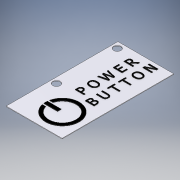
# Autodesk Inventor part: Power Button Plate
Saved by Autodesk Inventor 2019 (Build 230136000, 136)
## iProperties
Created: 2019-02-07
Part Number: Power Button Plate
Material: Generic
Document SubType Name: Modeling
Designer: mrhftc
Density: 1 g/cm^3
Appearance: Default
Author: mrhftc
Autodesk Inventor part; units mm, degrees
ref_plane "YZ Plane" through (0, 0, 0) normal (1, 0, 0) x (0, 1, 0)
ref_plane "XZ Plane" through (0, 0, 0) normal (0, 1, 0) x (-1, 0, 0)
ref_plane "XY Plane" through (0, 0, 0) normal (0, 0, 1) x (1, 0, 0)
sketch "Sketch1" plane through (0, 0, 0) normal (0, 1, 0) x (-1, 0, 0)
  line L0 (9.9313, 40.7784) -> (41.6813, 40.7784)
  line L1 (41.6813, 40.7784) -> (41.6813, 104.2784)
  line L2 (41.6813, 104.2784) -> (9.9313, 104.2784)
  line L3 (9.9313, 104.2784) -> (9.9313, 40.7784)
  point P0 (0, 0)
  dimension "d0" = 63.5
  dimension "d1" = 31.75
  constraints: 8 end point, 2 parallel, 1 horizontal, 1 perpendicular
  measures "d0" distance between parallel lines of L0 L2
  measures "d1" distance between parallel lines of L3 L1
extrude "Extrusion1" add sketch "Sketch1" along normal blind 0.3175
sketch "Sketch2" plane through (0, 0.3175, 0) normal (0, 1, 0) x (1, 0, 0)
  line L0 (-9.9313, -40.7784) -> (-41.6813, -40.7784) construction
  line L1 (-41.6813, -40.7784) -> (-41.6813, -104.2784) construction
  line L2 (-9.9313, -104.2784) -> (-9.9313, -40.7784) construction
  line L3 (-9.9313, -104.2784) -> (-35.3313, -104.2784)
  line L4 (-35.3313, -104.2784) -> (-35.3313, -40.7784)
  line L5 (-35.3313, -40.7784) -> (-9.9313, -40.7784)
  line L6 (-9.9313, -40.7784) -> (-9.9313, -104.2784)
  circle A0 centre (-38.5063, -44.3234) radius 2.1
  circle A1 centre (-38.5063, -78.8784) radius 2.1
  arc A2 (-32.0131, -93.4738) -> (-32.0131, -89.3044) centre (-22.6313, -91.3891) ccw
  arc A3 (-30.0496, -93.4738) -> (-30.0496, -89.3044) centre (-22.6313, -91.3891) ccw
  line L7 (-32.2013, -92.4142) -> (-24.3428, -92.4142)
  line L8 (-24.3428, -92.4142) -> (-24.3428, -90.3641)
  line L9 (-24.3428, -90.3641) -> (-32.2013, -90.3641)
  line L10 (-32.2013, -90.3641) -> (-32.2013, -92.4142)
  line L11 (-32.0131, -93.4738) -> (-30.0496, -93.4738)
  line L12 (-32.0131, -89.3044) -> (-30.0496, -89.3044)
  line L13 (-31.0313, -79.4258) -> (-24.997, -79.4258)
  line L14 (-24.997, -79.4258) -> (-24.997, -43.023)
  line L15 (-24.997, -43.023) -> (-31.0313, -43.023)
  line L16 (-31.0313, -43.023) -> (-31.0313, -79.4258)
  spline S0 degree 2 poles (-28.5456, -73.5374) (-28.2163, -73.5374) (-27.6235, -73.7721) (-27.4176, -73.982) knots 0 0 0 1 2 2 2
  spline S1 degree 2 poles (-27.4176, -73.982) (-27.1583, -74.2455) (-26.8907, -74.9577) (-26.8907, -75.5011) knots 0 0 0 1 2 2 2
  line L17 (-26.8907, -75.5011) -> (-26.8907, -76.0733)
  line L18 (-26.8907, -76.0733) -> (-24.997, -76.0733)
  line L19 (-24.997, -76.0733) -> (-24.997, -76.7485)
  line L20 (-24.997, -76.7485) -> (-30.077, -76.7485)
  line L21 (-30.077, -76.7485) -> (-30.077, -75.4723)
  spline S2 degree 2 poles (-30.077, -75.4723) (-30.077, -75.0194) (-29.9288, -74.3855) (-29.76, -74.1426) knots 0 0 0 1 2 2 2
  spline S3 degree 2 poles (-29.76, -74.1426) (-29.5665, -73.8585) (-28.9696, -73.5374) (-28.5456, -73.5374) knots 0 0 0 1 2 2 2
  spline S4 degree 2 poles (-28.525, -74.2414) (-28.7885, -74.2414) (-29.1754, -74.4225) (-29.2989, -74.6078) knots 0 0 0 1 2 2 2
  spline S5 degree 2 poles (-29.2989, -74.6078) (-29.406, -74.7683) (-29.4924, -75.1965) (-29.4924, -75.5134) knots 0 0 0 1 2 2 2
  line L22 (-29.4924, -75.5134) -> (-29.4924, -76.0733)
  line L23 (-29.4924, -76.0733) -> (-27.467, -76.0733)
  line L24 (-27.467, -76.0733) -> (-27.467, -75.6122)
  spline S6 degree 2 poles (-27.467, -75.6122) (-27.467, -75.2006) (-27.5988, -74.6942) (-27.7717, -74.5296) knots 0 0 0 1 2 2 2
  spline S7 degree 2 poles (-27.7717, -74.5296) (-27.924, -74.3772) (-28.2821, -74.2414) (-28.525, -74.2414) knots 0 0 0 1 2 2 2
  spline S8 degree 2 poles (-29.4965, -67.1195) (-29.159, -66.8313) (-28.171, -66.5102) (-27.537, -66.5102) knots 0 0 0 1 2 2 2
  spline S9 degree 2 poles (-27.537, -66.5102) (-26.9195, -66.5102) (-25.9191, -66.8231) (-25.5816, -67.1195) knots 0 0 0 1 2 2 2
  spline S10 degree 2 poles (-25.5816, -67.1195) (-25.2275, -67.4324) (-24.89, -68.2598) (-24.89, -68.758) knots 0 0 0 1 2 2 2
  spline S11 degree 2 poles (-24.89, -68.758) (-24.89, -69.2725) (-25.2399, -70.0959) (-25.5816, -70.3964) knots 0 0 0 1 2 2 2
  spline S12 degree 2 poles (-25.5816, -70.3964) (-25.9191, -70.6887) (-26.9113, -71.0016) (-27.537, -71.0016) knots 0 0 0 1 2 2 2
  spline S13 degree 2 poles (-27.537, -71.0016) (-28.1751, -71.0016) (-29.1466, -70.6846) (-29.4965, -70.3923) knots 0 0 0 1 2 2 2
  spline S14 degree 2 poles (-29.4965, -70.3923) (-29.8341, -70.0959) (-30.184, -69.2684) (-30.184, -68.758) knots 0 0 0 1 2 2 2
  spline S15 degree 2 poles (-30.184, -68.758) (-30.184, -68.2392) (-29.8218, -67.4077) (-29.4965, -67.1195) knots 0 0 0 1 2 2 2
  spline S16 degree 2 poles (-27.537, -67.2142) (-28.0392, -67.2142) (-28.8173, -67.4324) (-29.0725, -67.63) knots 0 0 0 1 2 2 2
  spline S17 degree 2 poles (-29.0725, -67.63) (-29.336, -67.8317) (-29.5995, -68.3998) (-29.5995, -68.7538) knots 0 0 0 1 2 2 2
  spline S18 degree 2 poles (-29.5995, -68.7538) (-29.5995, -69.1202) (-29.3442, -69.6719) (-29.0725, -69.8818) knots 0 0 0 1 2 2 2
  spline S19 degree 2 poles (-29.0725, -69.8818) (-28.8132, -70.0835) (-28.031, -70.2976) (-27.537, -70.2976) knots 0 0 0 1 2 2 2
  spline S20 degree 2 poles (-27.537, -70.2976) (-26.5366, -70.2976) (-25.4745, -69.4578) (-25.4745, -68.7538) knots 0 0 0 1 2 2 2
  spline S21 degree 2 poles (-25.4745, -68.7538) (-25.4745, -68.0499) (-26.5366, -67.2142) (-27.537, -67.2142) knots 0 0 0 1 2 2 2
  line L25 (-30.077, -57.894) -> (-24.997, -59.1702)
  line L26 (-24.997, -59.1702) -> (-24.997, -59.9276)
  line L27 (-24.997, -59.9276) -> (-29.2125, -60.9609)
  line L28 (-29.2125, -60.9609) -> (-24.997, -61.9654)
  line L29 (-24.997, -61.9654) -> (-24.997, -62.7146)
  line L30 (-24.997, -62.7146) -> (-30.077, -64.0114)
  line L31 (-30.077, -64.0114) -> (-30.077, -63.3157)
  line L32 (-30.077, -63.3157) -> (-25.8656, -62.2947)
  line L33 (-25.8656, -62.2947) -> (-30.077, -61.282)
  line L34 (-30.077, -61.282) -> (-30.077, -60.5945)
  line L35 (-30.077, -60.5945) -> (-25.8162, -59.5736)
  line L36 (-25.8162, -59.5736) -> (-30.077, -58.5568)
  line L37 (-30.077, -58.5568) -> (-30.077, -57.894)
  line L38 (-24.997, -55.107) -> (-30.077, -55.107)
  line L39 (-30.077, -55.107) -> (-30.077, -51.9289)
  line L40 (-30.077, -51.9289) -> (-29.476, -51.9289)
  line L41 (-29.476, -51.9289) -> (-29.476, -54.4319)
  line L42 (-29.476, -54.4319) -> (-28.0845, -54.4319)
  line L43 (-28.0845, -54.4319) -> (-28.0845, -52.0977)
  line L44 (-28.0845, -52.0977) -> (-27.4835, -52.0977)
  line L45 (-27.4835, -52.0977) -> (-27.4835, -54.4319)
  line L46 (-27.4835, -54.4319) -> (-25.598, -54.4319)
  line L47 (-25.598, -54.4319) -> (-25.598, -51.9289)
  line L48 (-25.598, -51.9289) -> (-24.997, -51.9289)
  line L49 (-24.997, -51.9289) -> (-24.997, -55.107)
  line L50 (-24.997, -45.0746) -> (-24.997, -45.9515)
  line L51 (-24.997, -45.9515) -> (-27.0183, -47.557)
  line L52 (-27.0183, -47.557) -> (-27.0183, -48.3309)
  line L53 (-27.0183, -48.3309) -> (-24.997, -48.3309)
  line L54 (-24.997, -48.3309) -> (-24.997, -49.0061)
  line L55 (-24.997, -49.0061) -> (-30.077, -49.0061)
  line L56 (-30.077, -49.0061) -> (-30.077, -47.6969)
  spline S22 degree 2 poles (-30.077, -47.6969) (-30.077, -47.2606) (-29.9823, -46.6719) (-29.8094, -46.4043) knots 0 0 0 1 2 2 2
  spline S23 degree 2 poles (-29.8094, -46.4043) (-29.6365, -46.1367) (-29.0972, -45.828) (-28.6979, -45.828) knots 0 0 0 1 2 2 2
  spline S24 degree 2 poles (-28.6979, -45.828) (-28.1422, -45.828) (-27.3888, -46.3961) (-27.2077, -46.8818) knots 0 0 0 1 2 2 2
  line L57 (-27.2077, -46.8818) -> (-24.997, -45.0746)
  spline S25 degree 2 poles (-28.6444, -46.5319) (-28.8667, -46.5319) (-29.2084, -46.6884) (-29.3195, -46.853) knots 0 0 0 1 2 2 2
  spline S26 degree 2 poles (-29.3195, -46.853) (-29.4142, -46.9971) (-29.4924, -47.38) (-29.4924, -47.6599) knots 0 0 0 1 2 2 2
  line L58 (-29.4924, -47.6599) -> (-29.4924, -48.3309)
  line L59 (-29.4924, -48.3309) -> (-27.5823, -48.3309)
  line L60 (-27.5823, -48.3309) -> (-27.5823, -47.7381)
  spline S27 degree 2 poles (-27.5823, -47.7381) (-27.5823, -47.4458) (-27.6852, -46.9806) (-27.8458, -46.8201) knots 0 0 0 1 2 2 2
  spline S28 degree 2 poles (-27.8458, -46.8201) (-27.9857, -46.6719) (-28.3809, -46.5319) (-28.6444, -46.5319) knots 0 0 0 1 2 2 2
  spline S29 degree 2 poles (-18.1683, -75.9519) (-17.7896, -75.9519) (-17.2091, -76.24) (-17.0198, -76.4788) knots 0 0 0 1 2 2 2
  spline S30 degree 2 poles (-17.0198, -76.4788) (-16.7975, -76.767) (-16.6081, -77.4215) (-16.6081, -77.9402) knots 0 0 0 1 2 2 2
  line L61 (-16.6081, -77.9402) -> (-16.6081, -79.3975)
  line L62 (-16.6081, -79.3975) -> (-21.6881, -79.3975)
  line L63 (-21.6881, -79.3975) -> (-21.6881, -78.0514)
  spline S31 degree 2 poles (-21.6881, -78.0514) (-21.6881, -77.508) (-21.6181, -76.9646) (-21.4823, -76.7176) knots 0 0 0 1 2 2 2
  spline S32 degree 2 poles (-21.4823, -76.7176) (-21.3382, -76.4418) (-20.8648, -76.1906) (-20.5437, -76.1906) knots 0 0 0 1 2 2 2
  spline S33 degree 2 poles (-20.5437, -76.1906) (-20.1855, -76.1906) (-19.6174, -76.5694) (-19.4569, -76.9028) knots 0 0 0 1 2 2 2
  line L64 (-19.4569, -76.9028) -> (-19.4322, -76.9028)
  spline S34 degree 2 poles (-19.4322, -76.9028) (-19.3086, -76.45) (-18.6541, -75.9519) (-18.1683, -75.9519) knots 0 0 0 1 2 2 2
  spline S35 degree 2 poles (-18.1395, -76.6558) (-18.4277, -76.6558) (-18.7982, -76.8205) (-18.9299, -77.0675) knots 0 0 0 1 2 2 2
  spline S36 degree 2 poles (-18.9299, -77.0675) (-19.0122, -77.2281) (-19.0616, -77.6068) (-19.0616, -77.9567) knots 0 0 0 1 2 2 2
  line L65 (-19.0616, -77.9567) -> (-19.0616, -78.7224)
  line L66 (-19.0616, -78.7224) -> (-17.1844, -78.7224)
  line L67 (-17.1844, -78.7224) -> (-17.1844, -78.1749)
  spline S37 degree 2 poles (-17.1844, -78.1749) (-17.1844, -77.7303) (-17.2668, -77.2198) (-17.3985, -77.0222) knots 0 0 0 1 2 2 2
  spline S38 degree 2 poles (-17.3985, -77.0222) (-17.5344, -76.8328) (-17.8719, -76.6558) (-18.1395, -76.6558) knots 0 0 0 1 2 2 2
  spline S39 degree 2 poles (-20.449, -76.8946) (-20.6301, -76.8946) (-20.9018, -77.0181) (-20.98, -77.1539) knots 0 0 0 1 2 2 2
  spline S40 degree 2 poles (-20.98, -77.1539) (-21.0706, -77.3186) (-21.1118, -77.7179) (-21.1118, -78.0761) knots 0 0 0 1 2 2 2
  line L68 (-21.1118, -78.0761) -> (-21.1118, -78.7224)
  line L69 (-21.1118, -78.7224) -> (-19.6256, -78.7224)
  line L70 (-19.6256, -78.7224) -> (-19.6256, -77.9567)
  spline S41 degree 2 poles (-19.6256, -77.9567) (-19.6256, -77.6397) (-19.6915, -77.3392) (-19.7944, -77.1787) knots 0 0 0 1 2 2 2
  spline S42 degree 2 poles (-19.7944, -77.1787) (-19.8932, -77.0222) (-20.2102, -76.8946) (-20.449, -76.8946) knots 0 0 0 1 2 2 2
  spline S43 degree 2 poles (-16.5011, -71.3247) (-16.5011, -71.7734) (-16.7357, -72.4403) (-16.9704, -72.675) knots 0 0 0 1 2 2 2
  spline S44 degree 2 poles (-16.9704, -72.675) (-17.2338, -72.9426) (-17.9748, -73.1608) (-18.5182, -73.1608) knots 0 0 0 1 2 2 2
  line L71 (-18.5182, -73.1608) -> (-21.6881, -73.1608)
  line L72 (-21.6881, -73.1608) -> (-21.6881, -72.4856)
  line L73 (-21.6881, -72.4856) -> (-18.5182, -72.4856)
  spline S45 degree 2 poles (-18.5182, -72.4856) (-18.1642, -72.4856) (-17.6867, -72.3951) (-17.4932, -72.2674) knots 0 0 0 1 2 2 2
  spline S46 degree 2 poles (-17.4932, -72.2674) (-17.2874, -72.1316) (-17.0774, -71.6623) (-17.0774, -71.3247) knots 0 0 0 1 2 2 2
  spline S47 degree 2 poles (-17.0774, -71.3247) (-17.0774, -71.0077) (-17.2874, -70.5137) (-17.4932, -70.3779) knots 0 0 0 1 2 2 2
  spline S48 degree 2 poles (-17.4932, -70.3779) (-17.6867, -70.2503) (-18.1601, -70.1597) (-18.5018, -70.1597) knots 0 0 0 1 2 2 2
  line L74 (-18.5018, -70.1597) -> (-21.6881, -70.1597)
  line L75 (-21.6881, -70.1597) -> (-21.6881, -69.4845)
  line L76 (-21.6881, -69.4845) -> (-18.5182, -69.4845)
  spline S49 degree 2 poles (-18.5182, -69.4845) (-17.9872, -69.4845) (-17.2297, -69.6986) (-16.9704, -69.9703) knots 0 0 0 1 2 2 2
  spline S50 degree 2 poles (-16.9704, -69.9703) (-16.7316, -70.2132) (-16.5011, -70.8554) (-16.5011, -71.3247) knots 0 0 0 1 2 2 2
  line L77 (-16.6081, -65.1497) -> (-21.0871, -65.1497)
  line L78 (-21.0871, -65.1497) -> (-21.0871, -66.854)
  line L79 (-21.0871, -66.854) -> (-21.6881, -66.854)
  line L80 (-21.6881, -66.854) -> (-21.6881, -62.7702)
  line L81 (-21.6881, -62.7702) -> (-21.0871, -62.7702)
  line L82 (-21.0871, -62.7702) -> (-21.0871, -64.4745)
  line L83 (-21.0871, -64.4745) -> (-16.6081, -64.4745)
  line L84 (-16.6081, -64.4745) -> (-16.6081, -65.1497)
  line L85 (-16.6081, -58.8841) -> (-21.0871, -58.8841)
  line L86 (-21.0871, -58.8841) -> (-21.0871, -60.5884)
  line L87 (-21.0871, -60.5884) -> (-21.6881, -60.5884)
  line L88 (-21.6881, -60.5884) -> (-21.6881, -56.5046)
  line L89 (-21.6881, -56.5046) -> (-21.0871, -56.5046)
  line L90 (-21.0871, -56.5046) -> (-21.0871, -58.2089)
  line L91 (-21.0871, -58.2089) -> (-16.6081, -58.2089)
  line L92 (-16.6081, -58.2089) -> (-16.6081, -58.8841)
  spline S51 degree 2 poles (-21.1076, -50.2102) (-20.7701, -49.922) (-19.7821, -49.6009) (-19.1481, -49.6009) knots 0 0 0 1 2 2 2
  spline S52 degree 2 poles (-19.1481, -49.6009) (-18.5306, -49.6009) (-17.5302, -49.9138) (-17.1927, -50.2102) knots 0 0 0 1 2 2 2
  spline S53 degree 2 poles (-17.1927, -50.2102) (-16.8386, -50.5231) (-16.5011, -51.3505) (-16.5011, -51.8486) knots 0 0 0 1 2 2 2
  spline S54 degree 2 poles (-16.5011, -51.8486) (-16.5011, -52.3632) (-16.851, -53.1866) (-17.1927, -53.4871) knots 0 0 0 1 2 2 2
  spline S55 degree 2 poles (-17.1927, -53.4871) (-17.5302, -53.7794) (-18.5224, -54.0922) (-19.1481, -54.0922) knots 0 0 0 1 2 2 2
  spline S56 degree 2 poles (-19.1481, -54.0922) (-19.7862, -54.0922) (-20.7577, -53.7752) (-21.1076, -53.483) knots 0 0 0 1 2 2 2
  spline S57 degree 2 poles (-21.1076, -53.483) (-21.4452, -53.1866) (-21.7951, -52.3591) (-21.7951, -51.8486) knots 0 0 0 1 2 2 2
  spline S58 degree 2 poles (-21.7951, -51.8486) (-21.7951, -51.3299) (-21.4329, -50.4984) (-21.1076, -50.2102) knots 0 0 0 1 2 2 2
  spline S59 degree 2 poles (-19.1481, -50.3049) (-19.6503, -50.3049) (-20.4284, -50.5231) (-20.6836, -50.7207) knots 0 0 0 1 2 2 2
  spline S60 degree 2 poles (-20.6836, -50.7207) (-20.9471, -50.9224) (-21.2106, -51.4905) (-21.2106, -51.8445) knots 0 0 0 1 2 2 2
  spline S61 degree 2 poles (-21.2106, -51.8445) (-21.2106, -52.2109) (-20.9553, -52.7625) (-20.6836, -52.9725) knots 0 0 0 1 2 2 2
  spline S62 degree 2 poles (-20.6836, -52.9725) (-20.4243, -53.1742) (-19.6421, -53.3883) (-19.1481, -53.3883) knots 0 0 0 1 2 2 2
  spline S63 degree 2 poles (-19.1481, -53.3883) (-18.1477, -53.3883) (-17.0856, -52.5485) (-17.0856, -51.8445) knots 0 0 0 1 2 2 2
  spline S64 degree 2 poles (-17.0856, -51.8445) (-17.0856, -51.1406) (-18.1477, -50.3049) (-19.1481, -50.3049) knots 0 0 0 1 2 2 2
  line L93 (-16.6081, -43.043) -> (-16.6081, -43.8005)
  line L94 (-16.6081, -43.8005) -> (-20.9883, -46.0482)
  line L95 (-20.9883, -46.0482) -> (-16.6081, -46.0482)
  line L96 (-16.6081, -46.0482) -> (-16.6081, -46.6781)
  line L97 (-16.6081, -46.6781) -> (-21.6881, -46.6781)
  line L98 (-21.6881, -46.6781) -> (-21.6881, -45.7189)
  line L99 (-21.6881, -45.7189) -> (-17.6661, -43.6729)
  line L100 (-17.6661, -43.6729) -> (-21.6881, -43.6729)
  line L101 (-21.6881, -43.6729) -> (-21.6881, -43.043)
  line L102 (-21.6881, -43.043) -> (-16.6081, -43.043)
  point P0 (0, 0)
  dimension "d4" = 25.4
  dimension "d5" = 3.175
  dimension "d6" = 4.2
  dimension "d7" = 38.1
  dimension "d8" = 1.905
  constraints: 28 end point, 8 parallel, 4 centre point, 4 point on circle, 3 horizontal, 3 perpendicular, 1 coincident, 1 point on line, 1 vertical
  measures "d4" distance between parallel lines of L2 L4
  measures "d5" distance from line of L1 A0.centre
  measures "d6" diameter of A0
  measures "d7" distance from line of L0 A1.centre
  measures "d8" radial gap between concentric circles of A2 A3
extrude "Extrusion2" add sketch "Sketch2" along normal blind 0.254 contours A0 | A1 | L11 A3 L12 A2 | L10 L9 L8 L7 | L20 L21 S2 S3 S0 S1 L17 L18 L14 | L14 L51 L52 L53 L55 L56 S22 S23 S24 L57 | S11 S12 S13 S14 S15 S8 S9 S10 L14 | L14 S10 S11 | L30 L31 L32 L33 L34 L35 L36 L37 L25 L14 L27 L28 | L14 L38 L39 L40 L41 L42 L43 L44 L45 L46 L47 L48 | S29 S30 L61 L62 L63 S31 S32 S33 L64 S34 | S43 S44 L71 L72 L73 S45 S46 S47 S48 L74 L75 L76 S49 S50 | L77 L78 L79 L80 L81 L82 L83 L84 | L85 L86 L87 L88 L89 L90 L91 L92 | S51 S52 S53 S54 S55 S56 S57 S58 | L93 L94 L95 L96 L97 L98 L99 L100 L101 L102
sketch "Sketch3" plane through (0, 0.3175, 0) normal (0, 1, 0) x (1, 0, 0)
  circle A0 centre (-38.5063, -78.8784) radius 2.1 construction
  circle A1 centre (-38.5063, -44.3234) radius 2.1 construction
  circle A2 centre (-38.5063, -78.8784) radius 2.1
  circle A3 centre (-38.5063, -44.3234) radius 2.1
  point P0 (0, 0)
  constraints: 2 centre point, 2 coincident, 2 concentric
extrude "Extrusion3" add sketch "Sketch3" against normal blind 2.54
sketch "Sketch5" plane through (-38.5063, -2.2225, 44.3234) normal (0, -1, 0) x (1, 0, 0)
  circle A0 centre (0, 0) radius 2.1 construction
  circle A1 centre (0, 0) radius 2.1
  circle A2 centre (0, 34.5585) radius 2.1211
  point P0 (38.5063, -44.3234)
  constraints: 2 centre point, 1 coincident, 1 concentric
extrude "Extrusion4" cut sketch "Sketch5" against normal through all
body "Solid1"
